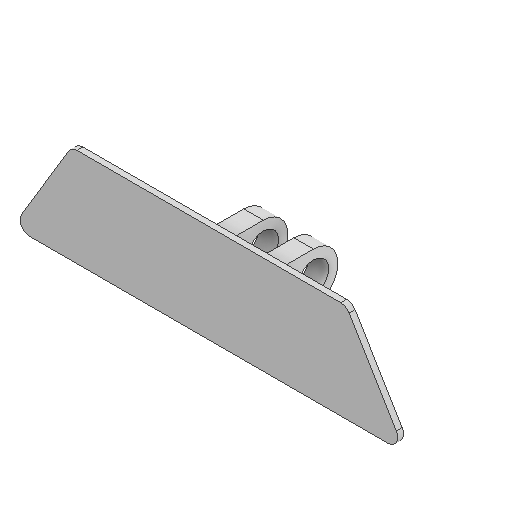
# Autodesk Inventor part: Lower Back Plate
Saved by Autodesk Inventor 2024 (Build 280153000, 153)
## iProperties
Created: 2025-04-26
Part Number: Lower Back Plate
Material: Generic
Document SubType Name: Modeling
Designer: Binara
Density: 1 g/cm^3
Appearance: Default
Author: Binara
Autodesk Inventor part; units mm, degrees
ref_plane "YZ Plane" through (0, 0, 0) normal (1, 0, 0) x (0, 1, 0)
ref_plane "XZ Plane" through (0, 0, 0) normal (0, 1, 0) x (-1, 0, 0)
ref_plane "XY Plane" through (0, 0, 0) normal (0, 0, 1) x (1, 0, 0)
sketch "Sketch1" plane through (0, 0, 0) normal (0, 0, 1) x (1, 0, 0)
  line L0 (0, 31.3291) -> (70, 31.3291)
  line L1 (70, 31.3291) -> (100, -18.6709)
  line L2 (100, -18.6709) -> (0, -18.6709)
  line L3 (0, 31.3291) -> (0, -18.6709)
  line L4 (0, 31.3291) -> (-70, 31.3291)
  line L5 (-70, 31.3291) -> (-100, -18.6709)
  line L6 (-100, -18.6709) -> (0, -18.6709)
  point P0 (0, 0)
  dimension "d0" = 100
  dimension "d1" = 70
  dimension "d2" = 50
  constraints: 14 end point, 2 symmetric about line, 1 horizontal, 1 parallel, 1 vertical, 1 vertical alignment
  measures "d0" distance of L1.end L2.end
  measures "d1" distance of L0.start L0.end
  measures "d2" distance between parallel lines of L2 L0
extrude "Extrusion1" add sketch "Sketch1" along normal blind 3
fillet "Fillet1" radius 5 4 edges at (70, 31.3291, 1.5) (100, -18.6709, 1.5) (-100, -18.6709, 1.5) (-70, 31.3291, 1.5)
sketch "Sketch2" plane through (0, 0, 0) normal (0, 0, -1) x (-1, 0, 0)
  line L0 (-17.75, -12.5) -> (17.75, -12.5)
  line L1 (17.75, -12.5) -> (17.75, 12.5)
  line L2 (17.75, 12.5) -> (-17.75, 12.5)
  line L3 (-17.75, 12.5) -> (-17.75, -12.5)
  line L4 (-17.75, -12.5) -> (17.75, 12.5) construction
  line L5 (17.75, -12.5) -> (-17.75, 12.5) construction
  line L6 (7.75, -12.5) -> (-7.75, -12.5)
  line L7 (-7.75, -12.5) -> (-7.75, 12.5)
  line L8 (-7.75, 12.5) -> (7.75, 12.5)
  line L9 (7.75, 12.5) -> (7.75, -12.5)
  line L10 (7.75, -12.5) -> (-7.75, 12.5) construction
  line L11 (-7.75, -12.5) -> (7.75, 12.5) construction
  point P0 (0, 0)
  dimension "d6" = 15.5
  dimension "d7" = 25
  dimension "d8" = 10
  constraints: 24 end point, 4 midpoint, 4 parallel, 2 horizontal, 2 perpendicular, 1 point on line
  measures "d6" distance between parallel lines of L7 L9
  measures "d7" distance of L0.end L1.end
  measures "d8" distance between parallel lines of L9 L1
extrude "Extrusion2" add sketch "Sketch2" along normal blind 45 contours L3 L2 L7 L0 | L9 L2 L1 L0
fillet "Fillet2" radius 12.5 4 edges at (12.75, 12.5, -45) (12.75, -12.5, -45) (-12.75, -12.5, -45) (-12.75, 12.5, -45)
sketch "Sketch3" plane through (17.75, -12.5, 0) normal (1, 0, 0) x (0, 0, -1)
  arc A0 (32.5, 0) -> (32.5, 25) centre (32.5, 12.5) ccw projected
  line L0 (0, 25) -> (32.5, 25) projected
  line L1 (0, 0) -> (0, 25) projected
  line L2 (0, 0) -> (32.5, 0) projected
  circle A1 centre (32.5, 12.5) radius 7.75
  point P0 (0, 12.5)
  dimension "d12" = 15.5
  constraints: 1 centre point, 1 coincident
  measures "d12" diameter of A1
extrude "Extrusion3" cut sketch "Sketch3" against normal up to surface (35.5 mm away) contours A1
body "Solid1"
